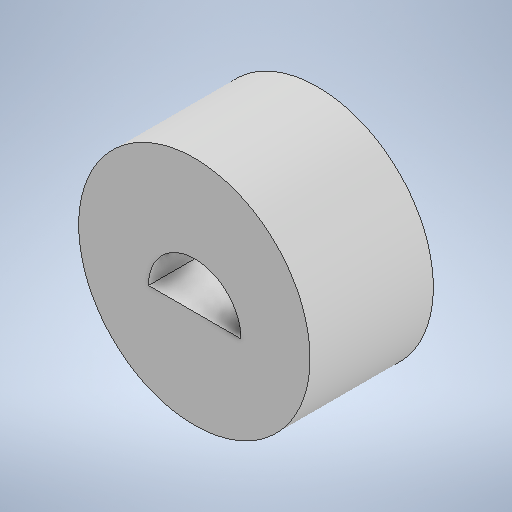
# Autodesk Inventor part: wheel
Saved by Autodesk Inventor 2025.3 (Build 293356030, 356C)
## iProperties
Created: 2026-06-23
Part Number: wheel
Material: Generic
Document SubType Name: Modeling
Designer: user
Density: 1 g/cm^3
Appearance: Default
Author: user
Autodesk Inventor part; units mm, degrees
ref_plane "YZ Plane" through (0, 0, 0) normal (1, 0, 0) x (0, 1, 0)
ref_plane "XZ Plane" through (0, 0, 0) normal (0, 1, 0) x (-1, 0, 0)
ref_plane "XY Plane" through (0, 0, 0) normal (0, 0, 1) x (1, 0, 0)
sketch "Sketch1" plane through (0, 0, 0) normal (0, 0, 1) x (1, 0, 0)
  circle A0 centre (0, 0) radius 37.5
  arc A1 (15.1278, -5.723) -> (-14.8722, -5.723) centre (0.1278, -5.723) ccw
  line L0 (-14.8722, -5.723) -> (15.1278, -5.723)
  dimension "d0" = 75
  dimension "d1" = 15
  constraints: 3 point on circle, 2 centre point, 2 end point, 1 coincident, 1 horizontal
  measures "d0" diameter of A0
  measures "d1" radius of A1
extrude "Extrusion1" add sketch "Sketch1" along normal blind 40
body "Solid1"
